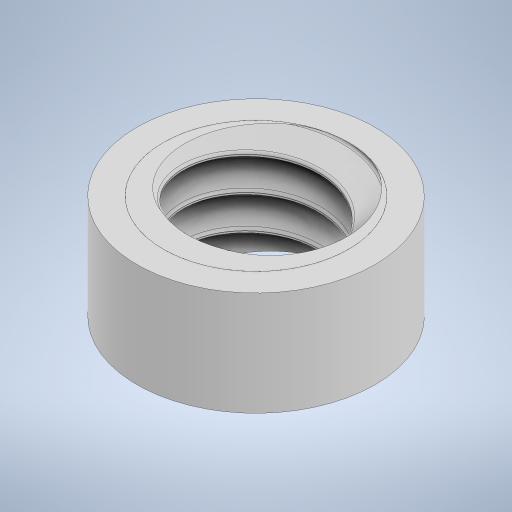
# Autodesk Inventor part: nut
Saved by Autodesk Inventor 2024 (Build 280153000, 153)
## iProperties
Created: 2023-09-15
Part Number: nut
Material: 일반
Document SubType Name: Modeling
Designer: jsw
Density: 1 g/cm^3
Appearance: 기본값
Author: jsw
Autodesk Inventor part; units mm, degrees
ref_plane "YZ Plane" through (0, 0, 0) normal (1, 0, 0) x (0, 1, 0)
ref_plane "XZ Plane" through (0, 0, 0) normal (0, 1, 0) x (-1, 0, 0)
ref_plane "XY Plane" through (0, 0, 0) normal (0, 0, 1) x (1, 0, 0)
sketch "스케치1" plane through (0, 0, 0) normal (0, 1, 0) x (-1, 0, 0)
  circle A0 centre (0, 0) radius 5.715
  circle A1 centre (0, 0) radius 4.445
  dimension "d0" = 11.43
  dimension "d1" = 8.89
  constraints: 2 centre point, 2 coincident
  measures "d0" diameter of A0
  measures "d1" diameter of A1
extrude "돌출1" add sketch "스케치1" along normal blind 5
thread "스레드2" size "3/8-16 UNC" class "2B" standard "ANSI Unified Screw Threads" full length
sketch "스케치5" plane through (0, 5, 0) normal (1, 0, 0) x (0, 0, 1)
  line L0 (4.445, 0) -> (4.445, 5)
  line L1 (4.445, 5) -> (3.2679, 5)
  line L2 (3.2679, 5) -> (3.2679, 0)
  line L3 (3.2679, 0) -> (4.445, 0)
  line L4 (0, -3.0773) -> (0, 6.3462) projected
  constraints: 8 end point
revolve "회전2" add sketch "스케치5" angle 360 about axis through (0, 5, 0) along (0, -1, 0) separate body
sketch "스케치4" plane through (0, 5, 4.445) normal (-1, 0, 0) x (0, -1, 0)
  line L0 (-0.9261, -0.0804) -> (-0.7939, -0.0804) construction
  line L1 (0.1322, -1.097) -> (-0.0001, -1.3511) construction
  line L2 (-1.5876, -1.3511) -> (-1.7199, -1.097) construction
  line L3 (-0.6616, -0.0804) -> (-0.7939, 0.1737) construction
  line L4 (-0.7939, 0.1737) -> (-0.9261, -0.0804) construction
  line L5 (-1.5876, -1.3511) -> (-1.4553, -1.097) construction
  line L6 (-0.6616, -0.0804) -> (-0.1324, -1.097)
  line L7 (-1.7199, -1.097) -> (-1.4553, -1.097) construction
  arc A0 (-1.7199, -1.097) -> (-1.5876, -1.1772) centre (-1.5876, -1.0281) ccw construction
  line L8 (0.1322, -1.097) -> (-0.1324, -1.097) construction
  line L9 (-1.5876, -1.3511) -> (-1.5876, -1.097) construction
  line L10 (-0.0001, -1.3511) -> (-0.0001, -1.097) construction
  line L11 (-0.7939, 0.1737) -> (-0.7939, -0.0002) construction
  line L12 (-1.5876, -1.1772) -> (-0.0001, -1.1772)
  arc A1 (-1.5876, -1.1772) -> (-1.4553, -1.097) centre (-1.5876, -1.0281) ccw
  line L13 (-0.1324, -1.097) -> (-0.0001, -1.3511) construction
  line L14 (-1.4553, -1.097) -> (-0.9261, -0.0804)
  line L15 (-0.0001, -0.0002) -> (-0.0001, 0.0177)
  line L16 (-0.0001, 0.0177) -> (-0.0001, -0.0002)
  line L17 (-0.0001, -0.0002) -> (0.0334, -0.0002)
  arc A2 (-0.1324, -1.097) -> (-0.0001, -1.1772) centre (-0.0001, -1.0281) ccw
  arc A3 (-0.0001, -1.1772) -> (0.1322, -1.097) centre (-0.0001, -1.0281) ccw construction
  arc A4 (-0.7939, -0.0002) -> (-0.9261, -0.0804) centre (-0.7939, -0.1493) ccw
  arc A5 (-0.6616, -0.0804) -> (-0.7939, -0.0002) centre (-0.7939, -0.1493) ccw
  line L18 (-0.7939, -0.0002) -> (-0.7939, -0.0804) construction
  line L19 (-0.7939, -0.0804) -> (-0.6616, -0.0804) construction
  dimension "d26" = 55
  dimension "d27" = 0.2541
  dimension "d28" = 0.2541
  dimension "d31" = 1.5875
  constraints: 40 end point, 12 point on circle, 10 parallel, 9 tangent, 7 collinear, 6 centre point, 2 midpoint, 2 point on line, 1 horizontal, 1 perpendicular, 4 other
  measures "d26" angle of L6 L14
  measures "d27" distance of L3.end L0.end
  measures "d28" distance of L1.end L10.end
  measures "d31" distance from line of L1.end L9
coil "코일2" sketch "스케치4" operation cut axis through (0, 5, 0) along (0, -1, 0) pitch 1.5891 turns 5.144462 hand right bodies 2
equation "\"d26\" = d33"
equation "\"d13\" = 55deg"
equation "\"d33\" = 55deg"
